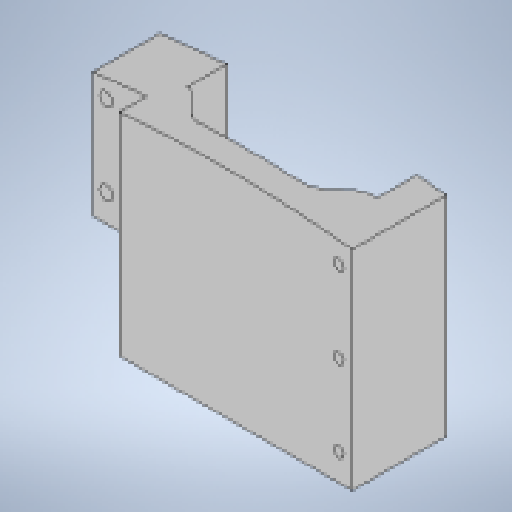
# Autodesk Inventor part: ReleaseMec2.0TopPlate
Saved by Autodesk Inventor 2025 (Build 290162000, 162)
## iProperties
Created: 2025-11-13
Part Number: ReleaseMec2.0TopPlate
Material: Generic
Document SubType Name: Modeling
Designer: ruven
Density: 1 g/cm^3
Appearance: Default
Author: ruven
Autodesk Inventor part; units mm, degrees
ref_plane "YZ Plane" through (0, 0, 0) normal (1, 0, 0) x (0, 1, 0)
ref_plane "XZ Plane" through (0, 0, 0) normal (0, 1, 0) x (-1, 0, 0)
ref_plane "XY Plane" through (0, 0, 0) normal (0, 0, 1) x (1, 0, 0)
sketch "Sketch1" plane through (0, 0, 0) normal (0, 0, 1) x (1, 0, 0)
  line L0 (-43.6429, 8.5714) -> (-63.6429, 8.5714)
  line L1 (-63.6429, 8.5714) -> (-63.6429, 18.5714)
  line L2 (-63.6429, 18.5714) -> (-28.6429, 18.5714)
  line L3 (-28.6429, 18.5714) -> (-28.6429, 8.5714)
  line L4 (-28.6429, 8.5714) -> (42.5571, 8.5714)
  line L5 (42.5571, 8.5714) -> (42.5571, -1.4286)
  line L6 (42.5571, -1.4286) -> (-43.6429, -1.4286)
  line L7 (-43.6429, -1.4286) -> (-43.6429, 8.5714)
  point P0 (0, 0)
  dimension "d0" = 10
  dimension "d1" = 10
  dimension "d2" = 20
  dimension "d3" = 86.2
  dimension "d4" = 15
  constraints: 16 end point, 4 parallel, 2 horizontal, 2 perpendicular
  measures "d0" distance between parallel lines of L2 L0
  measures "d1" distance of L0.start L6.end
  measures "d2" distance between parallel lines of L7 L1
  measures "d3" distance between parallel lines of L5 L7
  measures "d4" distance between parallel lines of L3 L7
extrude "Extrusion1" add sketch "Sketch1" along normal blind 80
chamfer "Chamfer1" distance 8 angle 45 1 edges at (-28.6429, 18.5714, 40)
fillet "Fillet1" radius 5 2 edges at (-36.6429, 18.5714, 40) (-28.6429, 8.5714, 40)
sketch "Sketch2" plane through (-63.6429, 18.5714, 80) normal (0, 1, 0) x (1, 0, 0)
  circle A0 centre (5, 10) radius 2.5
  circle A1 centre (5, 40) radius 2.5
  line L0 (24.9289, 0) -> (0, 0) projected
  line L1 (0, 80) -> (0, 0) projected
  line L2 (0, 80) -> (20, 80) projected
  line L3 (20, 80) -> (20, 0) projected
  line L4 (0, 80) -> (10, 80)
  line L5 (10, 80) -> (10, 50)
  line L6 (10, 50) -> (0, 50)
  line L7 (0, 50) -> (0, 80)
  point P0 (63.6429, 80)
  point P1 (20, 50)
  point P2 (0, 50)
  point P3 (10, 80)
  dimension "d11" = 10
  dimension "d12" = 40
  dimension "d13" = 5
  dimension "d14" = 5
  dimension "d15" = 5
  dimension "d16" = 5
  dimension "d31" = 10
  constraints: 8 end point, 2 centre point, 2 parallel, 1 horizontal, 1 perpendicular, 1 point on line
  measures "d11" distance from line of L0 A0.centre
  measures "d12" distance from line of L0 A1.centre
  measures "d13" distance from line of L1 A1.centre
  measures "d14" distance from line of L1 A0.centre
  measures "d15" diameter of A0
  measures "d16" diameter of A1
  measures "d31" distance from line of L6 A1.centre
extrude "Extrusion2" cut sketch "Sketch2" against normal blind 10 contours A0 | A1 | L1 L2 L5 L6
sketch "Sketch3" plane through (42.5571, 8.5714, 80) normal (0, 1, 0) x (1, 0, 0)
  circle A0 centre (-5, 10) radius 2
  circle A1 centre (-5, 40) radius 2
  circle A2 centre (-5, 70) radius 2
  line L0 (0, 80) -> (0, 0) projected
  line L1 (0, 80) -> (-67.2, 80) projected
  line L2 (0, 0) -> (-67.2, 0) projected
  point P0 (-42.5571, 80)
  dimension "d20" = 4
  dimension "d21" = 4
  dimension "d22" = 4
  dimension "d23" = 5
  dimension "d24" = 5
  dimension "d25" = 5
  dimension "d26" = 10
  dimension "d27" = 40
  dimension "d28" = 10
  constraints: 3 centre point
  measures "d20" diameter of A0
  measures "d21" diameter of A1
  measures "d22" diameter of A2
  measures "d23" distance from line of L0 A0.centre
  measures "d24" distance from line of L0 A1.centre
  measures "d25" distance from line of L0 A2.centre
  measures "d26" distance from line of L1 A2.centre
  measures "d27" distance from line of L1 A1.centre
  measures "d28" distance from line of L2 A0.centre
extrude "Extrusion3" cut sketch "Sketch3" against normal blind 10
sketch "Sketch4" plane through (42.5571, 8.5714, 80) normal (0, 1, 0) x (1, 0, 0)
  arc A0 (-125.8221, 5.2659) -> (2.953, 4.275) centre (-58.1, 438.1) ccw
  line L0 (0, 0) -> (-67.2, 0) projected
  line L1 (0, 80) -> (0, 0) projected
  line L2 (2.953, 4.275) -> (3.8116, -7.869)
  line L3 (3.8116, -7.869) -> (-122.3226, -7.869)
  line L4 (-122.3226, -7.869) -> (-125.8221, 5.2659)
  point P0 (-42.5571, 80)
  point P1 (0, 3.8696)
  point P2 (-58.1, 0)
  point P3 (-0.5169, 0)
  dimension "d32" = 876.2
  dimension "d33" = 0
  dimension "d34" = 58.1
  constraints: 6 end point, 2 point on circle, 1 centre point, 1 horizontal
  measures "d32" diameter of A0
  measures "d33" distance edge to line of A0 L0
  measures "d34" distance from line of A0.centre L1
extrude "Extrusion4" cut sketch "Sketch4" along normal through all both and the other way through all
sketch "Sketch5" plane through (-24.6429, 8.5714, 0) normal (0, 1, 0) x (1, 0, 0)
  circle A0 centre (62.2, -70) radius 2 projected
  circle A1 centre (62.2, -70) radius 2
  circle A2 centre (62.2, -40) radius 2 projected
  circle A3 centre (62.2, -40) radius 2
  circle A4 centre (62.2, -10) radius 2 projected
  circle A5 centre (62.2, -10) radius 2
  line L0 (67.2, 0) -> (67.2, -80) projected
  line L1 (67.2, -76.1304) -> (67.2, 0)
  line L2 (67.2, 0) -> (52.2, 0)
  line L3 (67.2, 0) -> (0, 0) projected
  line L4 (52.2, 0) -> (52.2, -77.8748)
  arc A6 (-19, -79.0979) -> (67.2, -76.1304) centre (9.1, 358.1) ccw projected
  arc A7 (-55.9, -73.5326) -> (94.1, -73.5326) centre (19.1, 358.0999) ccw projected
  arc A8 (-55.9, -73.5326) -> (94.1, -73.5326) centre (19.1, 358.0999) ccw projected
  arc A9 (-55.9, -73.5326) -> (94.1, -73.5326) centre (19.1, 358.0999) ccw projected
  circle A10 centre (-30.9, 438.0999) radius 2 projected
  circle A11 centre (-30.9, 308.0999) radius 2 projected
  circle A12 centre (69.1, 278.0999) radius 2 projected
  circle A13 centre (69.1, 308.0999) radius 2 projected
  circle A14 centre (69.1, 468.0999) radius 2 projected
  circle A15 centre (-30.9, 468.0999) radius 2 projected
  circle A16 centre (69.1, 408.0999) radius 2 projected
  circle A17 centre (-30.9, 248.0999) radius 2 projected
  circle A18 centre (69.1, 248.0999) radius 2 projected
  circle A19 centre (-30.9, 278.0999) radius 2 projected
  circle A20 centre (-30.9, 408.0999) radius 2 projected
  circle A21 centre (69.1, 438.0999) radius 2 projected
  circle A22 centre (-24, 756.1997) radius 2 projected
  circle A23 centre (62.2, -10) radius 2 projected
  circle A24 centre (62.2, -70) radius 2 projected
  circle A25 centre (-34, -40) radius 2.5 projected
  circle A26 centre (-24, 726.1997) radius 2 projected
  circle A27 centre (-24, 786.1997) radius 2 projected
  circle A28 centre (62.2, -40) radius 2 projected
  circle A29 centre (-34, -70) radius 2.5 projected
  circle A30 centre (72.2, 756.1997) radius 2.5 projected
  circle A31 centre (72.2, 786.1997) radius 2.5 projected
  circle A32 centre (-0.9, 338.0999) radius 2.5 projected
  circle A33 centre (39.1, 338.0999) radius 2.5 projected
  circle A34 centre (-0.9, 378.0999) radius 2.5 projected
  circle A35 centre (39.1, 378.0999) radius 2.5 projected
  circle A36 centre (19.1, 358.0999) radius 7.5 projected
  arc A37 (-55.9, -73.5326) -> (94.1, -73.5326) centre (19.1, 358.0999) ccw projected
  line L5 (94.1, -73.5326) -> (94.1, 789.7324) projected
  arc A38 (94.1, 789.7324) -> (-55.9, 789.7324) centre (19.1, 358.0999) ccw projected
  line L6 (-55.9, 789.7324) -> (-55.9, -73.5326) projected
  circle A39 centre (69.1, 158.0999) radius 2 projected
  circle A40 centre (-30.9, 38.0999) radius 2 projected
  circle A41 centre (69.1, 558.0999) radius 2 projected
  circle A42 centre (69.1, 518.0999) radius 2 projected
  circle A43 centre (-30.9, 638.0999) radius 2 projected
  circle A44 centre (69.1, 638.0999) radius 2 projected
  circle A45 centre (-30.9, 598.0999) radius 2 projected
  circle A46 centre (69.1, 118.0999) radius 2 projected
  circle A47 centre (-30.9, 118.0999) radius 2 projected
  circle A48 centre (69.1, 78.0999) radius 2 projected
  circle A49 centre (-30.9, 198.0999) radius 2 projected
  circle A50 centre (69.1, 198.0999) radius 2 projected
  circle A51 centre (-30.9, 678.0999) radius 2 projected
  circle A52 centre (-30.9, 558.0999) radius 2 projected
  circle A53 centre (69.1, 678.0999) radius 2 projected
  circle A54 centre (-30.9, 518.0999) radius 2 projected
  circle A55 centre (69.1, 598.0999) radius 2 projected
  circle A56 centre (69.1, 38.0999) radius 2 projected
  circle A57 centre (-30.9, 158.0999) radius 2 projected
  circle A58 centre (-30.9, 78.0999) radius 2 projected
  circle A59 centre (29.9074, 423.6249) radius 2 projected
  circle A60 centre (-0.0926, 473.6249) radius 2 projected
  circle A61 centre (-0.0926, 423.6249) radius 2 projected
  circle A62 centre (29.9074, 473.6249) radius 2 projected
  point P0 (24.6429, 0)
  point P1 (67.0008, -76.157)
  dimension "d37" = 15
  constraints: 6 end point, 3 centre point, 3 coincident, 1 collinear, 1 perpendicular, 1 point on circle, 1 point on line
  measures "d37" distance of L0.start L2.end
extrude "Extrusion5" add sketch "Sketch5" along normal blind 10 contours L0 A6 L4 L2
chamfer "Chamfer2" distance 10 angle 45 1 edges at (27.5571, 8.5714, 38.9374)
fillet "Fillet2" radius 10 3 edges at (17.5572, 8.5714, 39.3739) (27.5571, 18.5713, 38.9374) (27.5571, 18.5714, 38.9374)
sketch "Sketch6" plane through (-24.6429, 18.5714, 0) normal (0, 1, 0) x (1, 0, 0)
  circle A0 centre (62.2, -70) radius 2 projected
  circle A1 centre (62.2, -40) radius 2 projected
  circle A2 centre (62.2, -10) radius 2 projected
  line L0 (56.3421, -77.4454) -> (56.3421, 0) projected
  arc A3 (56.3421, -77.4454) -> (67.2, -76.1304) centre (9.1, 358.1) ccw projected
  line L1 (67.2, -76.1304) -> (67.2, 0) projected
  line L2 (67.2, 0) -> (56.3421, 0) projected
  circle A4 centre (-34, -70) radius 2.5 projected
  circle A5 centre (-34, -40) radius 2.5 projected
  arc A6 (-39, -77.3515) -> (-14.0711, -79.3868) centre (9.1, 358.1) ccw projected
  line L3 (-14.0711, 0) -> (-14.0711, -79.3868) projected
  line L4 (-14.0711, 0) -> (-29, 0) projected
  line L5 (-29, 0) -> (-29, -30) projected
  line L6 (-29, -30) -> (-39, -30) projected
  line L7 (-39, -30) -> (-39, -77.3515) projected
  point P0 (24.6429, 0)
extrude "Extrusion6" add sketch "Sketch6" along normal blind 14.8
body "Solid1"
